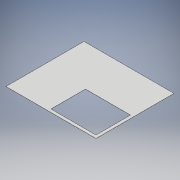
# Autodesk Inventor part: rightPanel
Saved by Autodesk Inventor 2017 (Build 210142000, 142)
## iProperties
Created: 2017-06-07
Part Number: rightPanel
Material: Generic
Document SubType Name: Sheet Metal
Designer: Roko
Density: 1 g/cm^3
Sheet Metal Rule: Default_mm
Appearance: Default
Author: Roko
Autodesk Inventor part; units mm, degrees
ref_plane "YZ Plane" through (0, 0, 0) normal (1, 0, 0) x (0, 1, 0)
ref_plane "XZ Plane" through (0, 0, 0) normal (0, 1, 0) x (-1, 0, 0)
ref_plane "XY Plane" through (0, 0, 0) normal (0, 0, 1) x (1, 0, 0)
sketch "Sketch1" plane through (0, 0, 0) normal (0, 0, 1) x (1, 0, 0)
  line L0 (-150, -130) -> (150, -130)
  line L1 (150, -130) -> (150, 130)
  line L2 (150, 130) -> (-150, 130)
  line L3 (-150, 130) -> (-150, -130)
  line L4 (-150, -130) -> (150, 130) construction
  line L5 (150, -130) -> (-150, 130) construction
  point P0 (0, 0)
  dimension "d0" = 300
  dimension "d1" = 260
  measures "d0" distance of L2.end L1.end
  measures "d1" distance of L1.end L0.end
extrude "Plate1" add sketch "Sketch1" along normal blind 0.5
sketch "Sketch3" plane through (0, 0, 0.5) normal (0, 0, 1) x (1, 0, 0)
  line L0 (-140, -120) -> (140, -120)
  line L1 (140, -120) -> (140, 120)
  line L2 (140, 120) -> (-140, 120)
  line L3 (-140, 120) -> (-140, -120)
  line L4 (-140, -120) -> (140, 120) construction
  line L5 (140, -120) -> (-140, 120) construction
  line L6 (140, -120) -> (-10, -120)
  line L7 (-10, -120) -> (-10, -5)
  line L8 (-10, -5) -> (140, -5)
  line L9 (140, -5) -> (140, -120)
  point P0 (0, 0)
  dimension "d3" = 280
  dimension "d4" = 240
  dimension "d5" = 150
  dimension "d6" = 115
  constraints: 20 end point, 4 parallel, 2 horizontal, 2 midpoint, 2 perpendicular
  measures "d3" distance of L2.end L1.end
  measures "d4" distance of L1.end L0.end
  measures "d5" distance of L7.end L8.end
  measures "d6" distance of L6.end L7.end
extrude "Cut1" cut sketch "Sketch3" against normal blind 0.5 contours L7 L8 L1 L0
equation "\"d7\" = Thickness"
equation "\"BendRadius\" = Thickness"
equation "\"BendReliefWidth\" = Thickness"
equation "\"BendReliefDepth\" = 0.5 * Thickness"
equation "\"CornerReliefSize\" = 4 * Thickness"
equation "\"MinimumRemnant\" = 2 * Thickness"
equation "\"TransitionRadius\" = BendRadius"
equation "\"JacobiRadiusSize\" = BendRadius"
equation "\"GapSize\" = Thickness"
equation "\"d2\" = BendRadius"
equation "\"Thickness\" = 0.5"
body "Solid1"
